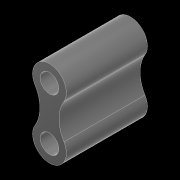
# Autodesk Inventor part: DriveTrainStandoffs
Saved by Autodesk Inventor 2022 (Build 260153000, 153)
## iProperties
Created: 2022-06-13
Part Number: DriveTrainStandoffs
Material: Custom TPU
Document SubType Name: Modeling
Designer: tandu
Density: 1.21 g/cm^3
Appearance: Smooth - Black
Author: tandu
Autodesk Inventor part; units mm, degrees
ref_plane "YZ Plane" through (0, 0, 0) normal (1, 0, 0) x (0, 1, 0)
ref_plane "XZ Plane" through (0, 0, 0) normal (0, 1, 0) x (-1, 0, 0)
ref_plane "Work Plane1" through (0, 0, 0) normal (0, 0, 1) x (1, 0, 0)
sketch "Sketch1" plane through (0, 0, 0) normal (0, 0, 1) x (1, 0, 0)
  circle A0 centre (0, 0) radius 1.75
  circle A1 centre (0, 0) radius 3.175
  circle A2 centre (0, 4.925) radius 3.175 construction
  circle A3 centre (0, 9.85) radius 1.75
  circle A4 centre (0, 9.85) radius 3.175
  arc A5 (2.7176, 8.2083) -> (2.7176, 1.6417) centre (8.1529, 4.925) ccw
  arc A6 (-2.7176, 1.6417) -> (-2.7176, 8.2083) centre (-8.1529, 4.925) ccw
  dimension "d0" = 6.35
  dimension "d3" = 3.5
  dimension "d5" = 6.35
  constraints: 8 point on circle, 7 centre point, 6 tangent, 4 equal radius, 3 coincident, 2 vertical alignment
  measures "d0" diameter of A1
  measures "d3" diameter of A0
  measures "d5" radius of A5
extrude "Extrusion1" add sketch "Sketch1" along normal blind 15.24
body "Solid1"
